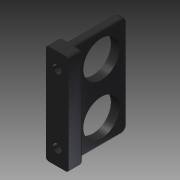
# Autodesk Inventor part: Sonar Mount
Saved by Autodesk Inventor 2015 (Build 190159000, 159)
## iProperties
Created: 2016-11-28
Part Number: Sonar Mount
Material: Generic
Document SubType Name: Modeling
Designer: James Yelland
Density: 1 g/cm^3
Appearance: Default
Author: James Yelland
Autodesk Inventor part; units mm, degrees
ref_plane "YZ Plane" through (0, 0, 0) normal (1, 0, 0) x (0, 1, 0)
ref_plane "XZ Plane" through (0, 0, 0) normal (0, 1, 0) x (-1, 0, 0)
ref_plane "XY Plane" through (0, 0, 0) normal (0, 0, 1) x (1, 0, 0)
sketch "Sketch1" plane through (0, 0, 0) normal (0, 1, 0) x (-1, 0, 0)
  line L0 (-4, 17.5) -> (-4, -17.5)
  line L1 (-4, -17.5) -> (4, -17.5)
  line L2 (4, -17.5) -> (4, 17.5)
  line L3 (4, 17.5) -> (-4, 17.5)
  line L4 (-4, 17.5) -> (4, -17.5) construction
  line L5 (-4, -17.5) -> (4, 17.5) construction
  line L6 (0, 0) -> (0, 8.89)
  line L7 (0, 0) -> (0, 12)
  circle A0 centre (0, 12) radius 1.45
  line L8 (0, 0) -> (0, -12)
  circle A1 centre (0, -12) radius 1.45
  dimension "d0" = 35
  dimension "d1" = 8
  dimension "d3" = 12
  dimension "d4" = 2.9
  dimension "d5" = 12
  dimension "d6" = 2.9
  constraints: 18 end point, 4 vertical, 2 centre point, 2 coincident, 2 midpoint, 2 parallel, 1 perpendicular
  measures "d0" distance of L0.start L0.end
  measures "d1" distance of L1.end L0.end
  measures "d3" distance of L6.start L7.end
  measures "d4" diameter of A0
  measures "d5" distance of L6.start L8.end
  measures "d6" diameter of A1
extrude "Extrusion1" add sketch "Sketch1" along normal blind 5
sketch "Sketch2" plane through (0, 5, 0) normal (0, 1, 0) x (1, 0, 0)
  line L0 (1.5, -17.5) -> (1.5, 17.5)
  line L1 (1.5, 17.5) -> (-1.5, 17.5)
  line L2 (-1.5, 17.5) -> (-1.5, -17.5)
  line L3 (-1.5, -17.5) -> (1.5, -17.5)
  line L4 (1.5, -17.5) -> (-1.5, 17.5) construction
  line L5 (1.5, 17.5) -> (-1.5, -17.5) construction
  point P0 (0, 0)
  dimension "d9" = 35
  dimension "d10" = 3
  constraints: 12 end point, 2 midpoint, 2 parallel, 1 perpendicular, 1 vertical
  measures "d9" distance of L0.start L0.end
  measures "d10" distance of L1.end L0.end
extrude "Extrusion2" add sketch "Sketch2" along normal blind 18
sketch "Sketch3" plane through (1.5, 5, 17.5) normal (1, 0, 0) x (0, 0, -1)
  line L0 (0, 18) -> (35, 18) projected
  line L1 (17.5, 18) -> (17.5, 9)
  line L2 (17.5, 18) -> (26.5, 18) construction
  line L3 (17.5, 9) -> (8.61, 9)
  line L4 (17.5, 9) -> (26.39, 9)
  line L5 (17.5, 9) -> (26.39, 9) construction
  circle A0 centre (8.61, 9) radius 6.35
  circle A1 centre (26.39, 9) radius 6.35
  point P0 (17.5, -5)
  dimension "d13" = 9
  dimension "d14" = 90
  dimension "d15" = 8.89
  dimension "d16" = 90
  dimension "d17" = 8.89
  dimension "d18" = 0
  dimension "d19" = 12.7
  dimension "d20" = 12.7
  constraints: 10 end point, 3 horizontal, 2 centre point, 2 coincident, 2 equal length, 1 midpoint, 1 perpendicular, 1 vertical
  measures "d13" distance of L1.start L1.end
  measures "d14" angle of L1 L2
  measures "d15" distance of L1.end L3.end
  measures "d16" angle of L1 L3
  measures "d17" distance of L1.end L4.end
  measures "d18" distance between parallel lines of L4 L5
  measures "d19" diameter of A0
  measures "d20" diameter of A1
extrude "Extrusion3" cut sketch "Sketch3" against normal blind 15
fillet "Fillet1" radius 2 2 edges at (0, 23, -17.5) (0, 23, 17.5)
fillet "Fillet2" radius 1 4 edges at (4, 2.5, -17.5) (-4, 2.5, -17.5) (4, 2.5, 17.5) (-4, 2.5, 17.5)
fillet "Fillet3" radius 0.75 10 edges at (1.5, 22.4142, -16.9142) (1.5, 13, -17.5) (1.5, 22.4142, 16.9142) (1.5, 13, 17.5) (1.5, 23, 0) (-1.5, 22.4142, 16.9142) (-1.5, 13, 17.5) (-1.5, 22.4142, -16.9142) (-1.5, 13, -17.5) (-1.5, 23, 0)
fillet "Fillet4" radius 0.75 6 edges at (3.7071, 5, -17.2071) (-3.7071, 5, -17.2071) (-4, 5, 0) (-3.7071, 5, 17.2071) (3.7071, 5, 17.2071) (4, 5, 0)
body "Solid1"
